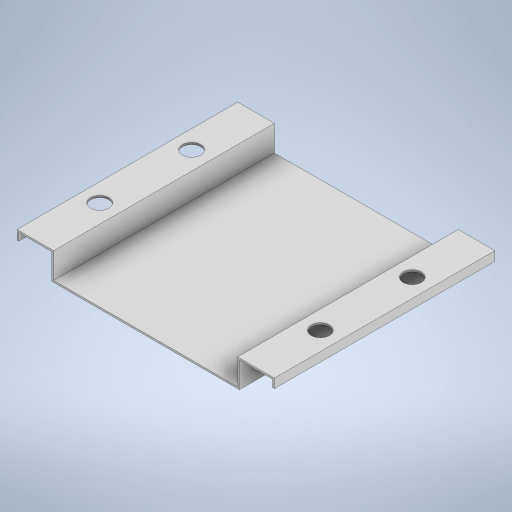
# Autodesk Inventor part: Pallet
Saved by Autodesk Inventor 2023 (Build 270158000, 158)
## iProperties
Created: 2023-02-09
Part Number: Pallet
Material: Generic
Document SubType Name: Modeling
Designer: HP
Density: 1 g/cm^3
Appearance: Default
Author: HP
Autodesk Inventor part; units mm, degrees
ref_plane "YZ Plane" through (0, 0, 0) normal (1, 0, 0) x (0, 1, 0)
ref_plane "XZ Plane" through (0, 0, 0) normal (0, 1, 0) x (-1, 0, 0)
ref_plane "XY Plane" through (0, 0, 0) normal (0, 0, 1) x (1, 0, 0)
sketch "Sketch1" plane through (0, 0, 0) normal (0, 0, 1) x (1, 0, 0)
  line L0 (0, 0) -> (0, 1)
  line L1 (0, 1) -> (0, 15)
  line L2 (0, 15) -> (20, 15)
  line L3 (20, 15) -> (20, 10)
  line L4 (20, 10) -> (19, 10)
  line L5 (19, 10) -> (19, 14)
  line L6 (19, 14) -> (1, 14)
  line L7 (1, 14) -> (1, 0)
  line L8 (1, 0) -> (-101, 0)
  line L9 (-101, 0) -> (-101, 14)
  line L10 (-101, 14) -> (-119, 14)
  line L11 (-119, 14) -> (-119, 10)
  line L12 (-119, 10) -> (-120, 10)
  line L13 (-120, 10) -> (-120, 15)
  line L14 (-120, 15) -> (-100, 15)
  line L15 (-100, 15) -> (-100, 1)
  line L16 (-100, 1) -> (0, 1)
  dimension "d1" = 14
  dimension "d2" = 20
  dimension "d3" = 5
  dimension "d4" = 1
  dimension "d5" = 4
  dimension "d6" = 18
  dimension "d7" = 102
  dimension "d8" = 14
  dimension "d9" = 18
  dimension "d10" = 4
  dimension "d11" = 1
  dimension "d12" = 5
  dimension "d13" = 20
  dimension "d14" = 14
  constraints: 34 end point, 7 point on line, 6 perpendicular, 2 parallel, 1 vertical
  measures "d1" distance of L0.end L1.end
  measures "d2" distance of L1.end L2.end
  measures "d3" distance of L2.end L3.end
  measures "d4" distance of L3.end L4.end
  measures "d5" distance of L4.end L5.end
  measures "d6" distance of L5.end L6.end
  measures "d7" distance of L7.end L8.end
  measures "d8" distance of L8.end L9.end
  measures "d9" distance of L9.end L10.end
  measures "d10" distance of L10.end L11.end
  measures "d11" distance of L11.end L12.end
  measures "d12" distance of L12.end L13.end
  measures "d13" distance of L13.end L14.end
  measures "d14" distance of L14.end L15.end
extrude "Extrusion1" add sketch "Sketch1" along normal blind 120
sketch "Sketch2" plane through (0, 15, 0) normal (0, 1, 0) x (1, 0, 0)
  circle A0 centre (10, -85) radius 5
  circle A1 centre (10, -35) radius 5
  circle A2 centre (-110, -35) radius 5
  circle A3 centre (-110, -85) radius 5
  line L0 (20, 0) -> (20, -120) projected
  line L1 (20, 0) -> (0, 0) projected
  line L2 (20, -120) -> (0, -120) projected
  line L3 (-120, 0) -> (-120, -120) projected
  dimension "d17" = 10
  dimension "d18" = 10
  dimension "d19" = 10
  dimension "d20" = 10
  constraints: 4 centre point
  measures "d17" diameter of A0
  measures "d18" diameter of A1
  measures "d19" diameter of A2
  measures "d20" diameter of A3
hole "Hole1" at (10, 15, 85) at (10, 15, 35) at (-110, 15, 35) at (-110, 15, 85) direction (0, -1, 0) diameter 10 end through all
body "Solid1"
